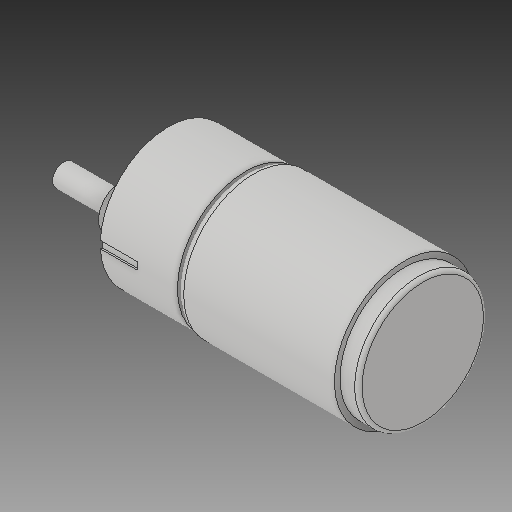
# Autodesk Inventor part: Двигатель
Saved by Autodesk Inventor 2018 (Build 220112000, 112)
## iProperties
Part Number: Двигатель
Material: Типовые
Document SubType Name: Modeling
Designer: sbnnl
Density: 1 g/cm^3
Appearance: По умолчанию
Author: sbnnl
Autodesk Inventor part; units mm, degrees
ref_plane "YZ Plane" through (0, 0, 0) normal (1, 0, 0) x (0, 1, 0)
ref_plane "XZ Plane" through (0, 0, 0) normal (0, 1, 0) x (-1, 0, 0)
ref_plane "XY Plane" through (0, 0, 0) normal (0, 0, 1) x (1, 0, 0)
sketch "Эскиз1" plane through (0, 0, 0) normal (1, 0, 0) x (0, 1, 0)
  circle A0 centre (0, 0) radius 18.5
  dimension "d0" = 37
  constraints: 1 centre point, 1 coincident
  measures "d0" diameter of A0
extrude "Выдавливание1" add sketch "Эскиз1" along normal blind 21
sketch "Эскиз2" plane through (21, 0, 0) normal (1, 0, 0) x (0, 0, -1)
  circle A0 centre (0, 0) radius 15
  dimension "d3" = 30
  constraints: 1 centre point, 1 coincident
  measures "d3" diameter of A0
extrude "Выдавливание2" add sketch "Эскиз2" along normal blind 0.2
sketch "Эскиз3" plane through (21.2, 0, 0) normal (1, 0, 0) x (0, 0, -1)
  circle A0 centre (0, 0) radius 19
  dimension "d6" = 38
  constraints: 1 centre point, 1 coincident
  measures "d6" diameter of A0
extrude "Выдавливание3" add sketch "Эскиз3" along normal blind 43
fillet "Сопряжение1" radius 2 1 edges at (21.2, 0, 19)
sketch "Эскиз4" plane through (64.2, 0, 0) normal (1, 0, 0) x (0, 0, -1)
  circle A0 centre (0, 0) radius 17.5
  dimension "d10" = 35
  constraints: 1 centre point, 1 coincident
  measures "d10" diameter of A0
extrude "Выдавливание4" add sketch "Эскиз4" along normal blind 5
fillet "Сопряжение2" radius 1 1 edges at (69.2, 0, 17.5)
sketch "Эскиз5" plane through (0, 0, 0) normal (-1, 0, 0) x (0, 0, 1)
  line L0 (0, 0) -> (27.1698, 0) construction
  circle A0 centre (7, 0) radius 6
  dimension "d14" = 12
  dimension "d15" = 7
  constraints: 2 end point, 1 centre point, 1 horizontal, 1 point on line
  measures "d14" diameter of A0
  measures "d15" distance of A0.centre L0.start
extrude "Выдавливание5" add sketch "Эскиз5" along normal blind 6
sketch "Эскиз6" plane through (-6, 0, 7) normal (-1, 0, 0) x (0, 0, 1)
  circle A0 centre (0, 0) radius 3
  circle A1 centre (0, 0) radius 6 projected
  point P0 (-7, 0)
  dimension "d18" = 6
  constraints: 1 centre point, 1 concentric
  measures "d18" diameter of A0
extrude "Выдавливание6" add sketch "Эскиз6" along normal blind 15.5 contours A0
sketch "Эскиз7" plane through (0, 0, 0) normal (-1, 0, 0) x (0, 0, 1)
  circle A0 centre (7, 0) radius 3 projected
  line L0 (0, 0) -> (22.9048, 0) construction
  line L1 (21, 1) -> (18, 1)
  line L2 (18, 1) -> (18, -1)
  line L3 (18, -1) -> (21, -1)
  line L4 (21, -1) -> (21, 1)
  dimension "d21" = 18
  dimension "d22" = 3
  dimension "d23" = 2
  constraints: 10 end point, 2 horizontal, 2 parallel, 1 perpendicular, 1 other
  measures "d21" distance from line of L2 L0.start
  measures "d22" distance between parallel lines of L4 L2
  measures "d23" distance between parallel lines of L3 L1
extrude "Выдавливание7" cut sketch "Эскиз7" against normal blind 10 contours L4 L3 L2 L1
